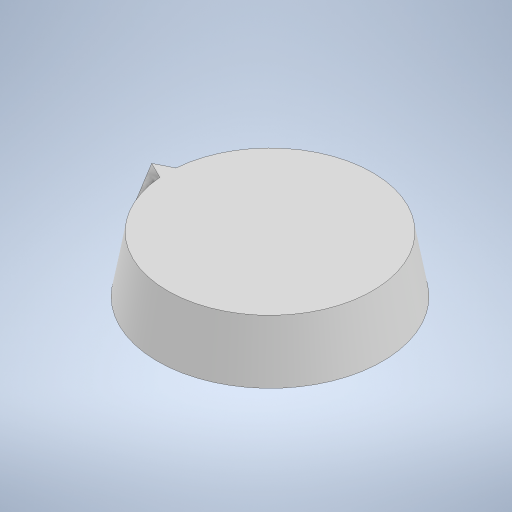
# Autodesk Inventor part: ChairDial(H)
Saved by Autodesk Inventor 2023 (Build 270158030, 158C)
## iProperties
Created: 2023-03-05
Part Number: ChairDial(H)
Material: Generic
Document SubType Name: Modeling
Designer: mpino
Density: 1 g/cm^3
Appearance: Default
Author: mpino
Autodesk Inventor part; units mm, degrees
ref_plane "YZ Plane" through (0, 0, 0) normal (1, 0, 0) x (0, 1, 0)
ref_plane "XZ Plane" through (0, 0, 0) normal (0, 1, 0) x (-1, 0, 0)
ref_plane "XY Plane" through (0, 0, 0) normal (0, 0, 1) x (1, 0, 0)
sketch "Sketch1" plane through (0, 0, 0) normal (0, 1, 0) x (-1, 0, 0)
  circle A0 centre (0, 0) radius 5.08
  line L0 (0, 0) -> (0, 3.175)
  line L1 (0, 0) -> (0, -3.175)
  circle A1 centre (0, 0) radius 6.35
  line L2 (0, 3.175) -> (6.35, 0)
  line L3 (0, -3.175) -> (6.35, 0)
  point P0 (5.037429, -0.656286)
  point P1 (5.037429, 0.656286)
  dimension "d3" = 12.7
  dimension "d0" = 10.16
  dimension "d1" = 3.175
  dimension "d2" = 3.175
  dimension "d4" = 6.35
  constraints: 8 end point, 2 coincident, 2 vertical, 1 centre point, 1 horizontal alignment, 2 other
  measures "d0" diameter of A0
  measures "d1" distance of L0.start L0.end
  measures "d2" distance of L0.start L1.end
  measures "d4" horizontal distance of L1.end L2.end
sketch "Sketch1 outline for Extrusion1" plane through (0, 0, 0) normal (0, 1, 0) x (-1, 0, 0)
  line L0 (5.037429, -0.656286) -> (6.35, 0)
  arc A0 (5.037429, 0.656286) -> (5.037429, -0.656286) centre (0, 0) ccw
  line L1 (6.35, 0) -> (5.037429, 0.656286)
extrude "Extrusion1" add sketch "Sketch1 outline for Extrusion1" along normal blind 2.54 draft -10
sketch "Sketch2" plane through (0, 0, 0) normal (0, -1, 0) x (1, 0, 0)
  circle A0 centre (0, 0) radius 1.27
  dimension "d7" = 2.54
  constraints: 1 centre point, 1 coincident
  measures "d7" diameter of A0
extrude "Extrusion2" cut sketch "Sketch2" against normal blind 1.27
body "Solid1"
